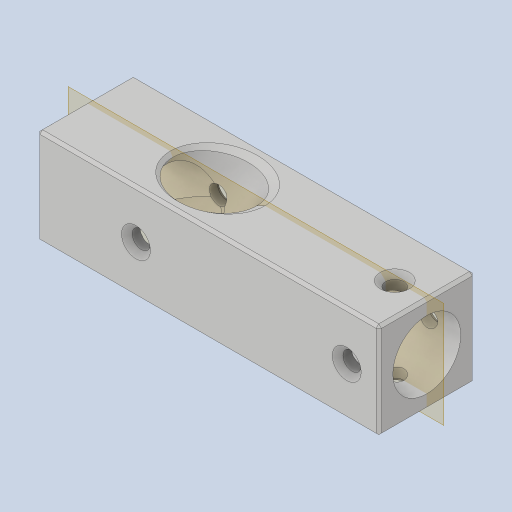
# Autodesk Inventor part: holderHolder
Saved by Autodesk Inventor 2024.1 (Build 281209000, 209)
## iProperties
Created: 2019-08-19
Part Number: holderHolder
Material: Generic
Document SubType Name: Modeling
Designer: Daniel
Density: 1 g/cm^3
Appearance: Default
Author: Daniel
Autodesk Inventor part; units mm, degrees
sketch "Sketch1" plane through (0, 0, 0) normal (0, 1, 0) x (-1, 0, 0)
  line L0 (0, 0) -> (-60, 0)
  line L1 (-60, 0) -> (-60, -18)
  line L2 (-60, -18) -> (0, -18)
  line L3 (0, -18) -> (0, 0)
  dimension "d0" = 60
  dimension "d1" = 18
  constraints: 8 end point, 2 parallel, 1 horizontal, 1 perpendicular
  measures "d0" distance of L1.end L2.end
  measures "d1" distance of L2.end L0.start
extrude "Extrusion1" add sketch "Sketch1" along normal blind 18
sketch "Sketch2" plane through (60, 0, 0) normal (1, 0, 0) x (0, 0, -1)
  line L0 (14.7, 6.639) -> (11.361, 3.3)
  line L1 (11.361, 3.3) -> (6.639, 3.3)
  line L2 (6.639, 3.3) -> (3.3, 6.639)
  line L3 (3.3, 6.639) -> (3.3, 11.361)
  line L4 (3.3, 11.361) -> (6.639, 14.7)
  line L5 (6.639, 14.7) -> (11.361, 14.7)
  line L6 (11.361, 14.7) -> (14.7, 11.361)
  line L7 (14.7, 11.361) -> (14.7, 6.639)
  line L8 (0, 18) -> (18, 18) construction
  line L9 (9, 18) -> (9, 0) construction
  line L10 (0, 0) -> (18, 0) construction
  line L11 (0, 0) -> (0, 18) construction
  line L12 (0, 9) -> (18, 9) construction
  line L13 (18, 0) -> (18, 18) construction
  point P0 (9, 9)
  dimension "d4" = 11.4
  dimension "d28" = 0
  constraints: 20 end point, 5 midpoint, 17 other
  measures "d4" distance between parallel lines of L1 L5
  measures "d28" angle of L12 L5
extrude "Extrusion2" cut sketch "Sketch2" against normal blind 18
sketch "Sketch3" plane through (42, 0, 0) normal (1, 0, 0) x (0, 0, -1)
  line L0 (14.7, 6.639) -> (11.361, 3.3) projected
  line L1 (14.7, 11.361) -> (14.7, 6.639) projected
  line L2 (11.361, 14.7) -> (14.7, 11.361) projected
  line L3 (6.639, 14.7) -> (11.361, 14.7) projected
  line L4 (3.3, 11.361) -> (6.639, 14.7) projected
  line L5 (3.3, 6.639) -> (3.3, 11.361) projected
  line L6 (6.639, 3.3) -> (3.3, 6.639) projected
  line L7 (11.361, 3.3) -> (6.639, 3.3) projected
  circle A0 centre (9, 9) radius 4
  point P0 (0, 0)
  dimension "d7" = 8
  constraints: 1 centre point
  measures "d7" diameter of A0
extrude "Extrusion3" cut sketch "Sketch3" against normal through all contours A0
sketch "Sketch4" plane through (0, 0, -18) normal (-1, 0, 0) x (0, 0, 1)
  circle A0 centre (9, 9) radius 4 projected
  circle A1 centre (9, 9) radius 6.5
  point P0 (18, 0)
  dimension "d10" = 13
  constraints: 1 centre point, 1 coincident
  measures "d10" diameter of A1
extrude "Extrusion4" cut sketch "Sketch4" against normal blind 20
ref_plane "Work Plane1" through (0, 0, -18) normal (-0.5735764, -0.819152, 0) x (0, 0, 1)
sketch "Sketch5" plane through (-5.043, 3.5311, 0) normal (0.5735764, 0.819152, 0) x (0.819152, -0.5735764, 0)
  circle A0 centre (16.1564, 9) radius 6.45
  line L0 (6.1564, 18) -> (6.1564, 0) construction
  line L1 (6.1564, 9) -> (16.1564, 9) construction
  dimension "d13" = 12.9
  dimension "d27" = 10
  constraints: 2 end point, 1 centre point, 1 horizontal, 1 midpoint
  measures "d13" diameter of A0
  measures "d27" distance from line of L0 L1.end
extrude "Extrusion5" cut sketch "Sketch5" along normal through all
ref_plane "Work Plane3" through (0, 0, -18) normal (0, -1, 0) x (0, 0, 1)
ref_plane "Work Plane2" through (42, -7.45, -11.361) normal (0, 1, 0) x (1, 0, 0)
sketch "Sketch9" plane through (60, 0, 0) normal (1, 0, 0) x (0, 0, -1)
  arc A0 (2.5812, 10.0241) -> (15.4188, 10.0241) centre (9, 9) ccw projected
  circle A1 centre (9, 9) radius 6
  line L0 (0, 0) -> (0, 18) projected
  line L1 (0, 18) -> (18, 18) projected
  line L2 (0, 0) -> (18, 0) projected
  line L3 (18, 0) -> (18, 18) projected
  dimension "d49" = 12
  constraints: 1 centre point, 1 coincident
  measures "d49" diameter of A1
extrude "Extrusion9" add sketch "Sketch9" along normal blind 4
sketch "Sketch6" plane through (0, 0, 0) normal (0, 0, 1) x (1, 0, 0)
  line L0 (0, 0) -> (0, 18) construction
  line L1 (0, 9) -> (48.5921, 9) construction
  circle A0 centre (18.5096, 9) radius 1.7
  line L2 (20.0817, 0) -> (4.3337, 0) projected
  line L3 (16.9375, 18) -> (32.6855, 18) projected
  line L4 (16.9375, 18) -> (20.0817, 0) construction
  line L5 (32.6855, 18) -> (4.3337, 0) construction
  dimension "d23" = 3.4
  constraints: 6 end point, 2 midpoint, 1 centre point, 1 point on line
  measures "d23" diameter of A0
extrude "Extrusion6" cut sketch "Sketch6" against normal through all
sketch "Sketch10" plane through (0, 0, -18) normal (0, -1, 0) x (0, 0, 1)
  circle A0 centre (9, -18.5096) radius 6.45
  line L0 (0, 0) -> (18, 0) projected
  line L1 (18, -16.8096) -> (18, -20.2096) projected
  point P0 (9, 0)
  point P1 (9, 0)
  point P2 (18, -18.5096)
  dimension "d59" = 12.9
  constraints: 3 midpoint, 2 vertical alignment, 1 centre point, 1 horizontal alignment
  measures "d59" diameter of A0
extrude "Extrusion10" [suppressed]
sketch "Sketch7" plane through (42, -7.45, -11.361) normal (0, 1, 0) x (1, 0, 0)
  circle A0 centre (16, -2.361) radius 1.7
  line L0 (18, -0.4875) -> (18, -4.2345) projected
  line L1 (18, 0) -> (0, 0) projected
  line L2 (0, 0) -> (0, -4.722) projected
  line L3 (18, -4.722) -> (0, -4.722) projected
  line L4 (18, 0) -> (18, -0.4875) projected
  line L5 (18, -4.2345) -> (18, -4.722) projected
  point P0 (-42, -11.361)
  dimension "d30" = 3.4
  dimension "d31" = 2.361
  dimension "d32" = 2.361
  dimension "d33" = 2
  constraints: 1 centre point
  measures "d30" diameter of A0
  measures "d31" distance from line of L1 A0.centre
  measures "d32" distance from line of L3 A0.centre
  measures "d33" distance from line of L0 A0.centre
extrude "Extrusion7" cut sketch "Sketch7" along normal through all contours A0
pattern_circular "Circular Pattern1" count 4 over 360 about axis through (60, 9, -9) along (1, 0, 0) of "Extrusion7"
ref_plane "Work Plane4" through (0, 0, -9) normal (0, 0, 1) x (1, 0, 0)
sketch "Sketch8" plane through (0, 0, 0) normal (0, -1, 0) x (1, 0, 0)
  line L0 (32, -18) -> (46, -18) construction
  line L1 (46, -18) -> (46, 0) construction
  line L2 (46, 0) -> (32, 0) construction
  line L3 (32, 0) -> (32, -18) construction
  line L4 (0, 0) -> (64, 0) projected
  line L5 (0, 0) -> (64, 0) projected
  line L6 (0, -18) -> (64, -18) projected
  circle A0 centre (58, -9) radius 1.7 projected
  spline S0 degree 2 poles (35.027, -5.8856) (35.027, -6.0832) (34.8862, -6.4389) (34.7602, -6.5624) knots 0 0 0 1 2 2 2
  spline S1 degree 2 poles (34.7602, -6.5624) (34.6021, -6.718) (34.1748, -6.8786) (33.8488, -6.8786) knots 0 0 0 1 2 2 2
  line L7 (33.8488, -6.8786) -> (33.5054, -6.8786)
  line L8 (33.5054, -6.8786) -> (33.5054, -8.0148)
  line L9 (33.5054, -8.0148) -> (33.1004, -8.0148)
  line L10 (33.1004, -8.0148) -> (33.1004, -4.9668)
  line L11 (33.1004, -4.9668) -> (33.8661, -4.9668)
  spline S2 degree 2 poles (33.8661, -4.9668) (34.1378, -4.9668) (34.5182, -5.0557) (34.6639, -5.157) knots 0 0 0 1 2 2 2
  spline S3 degree 2 poles (34.6639, -5.157) (34.8343, -5.2731) (35.027, -5.6312) (35.027, -5.8856) knots 0 0 0 1 2 2 2
  spline S4 degree 2 poles (34.6046, -5.898) (34.6046, -5.7399) (34.4959, -5.5077) (34.3848, -5.4336) knots 0 0 0 1 2 2 2
  spline S5 degree 2 poles (34.3848, -5.4336) (34.2884, -5.3694) (34.0316, -5.3175) (33.8414, -5.3175) knots 0 0 0 1 2 2 2
  line L12 (33.8414, -5.3175) -> (33.5054, -5.3175)
  line L13 (33.5054, -5.3175) -> (33.5054, -6.5328)
  line L14 (33.5054, -6.5328) -> (33.7821, -6.5328)
  spline S6 degree 2 poles (33.7821, -6.5328) (34.0291, -6.5328) (34.3329, -6.4537) (34.4317, -6.35) knots 0 0 0 1 2 2 2
  spline S7 degree 2 poles (34.4317, -6.35) (34.5231, -6.2586) (34.6046, -6.0437) (34.6046, -5.898) knots 0 0 0 1 2 2 2
  spline S8 degree 2 poles (36.1484, -5.2558) (36.0372, -5.2558) (35.8174, -5.3101) (35.7112, -5.3521) knots 0 0 0 1 2 2 2
  spline S9 degree 2 poles (35.7112, -5.3521) (35.6124, -5.3941) (35.4666, -5.483) (35.4098, -5.5225) knots 0 0 0 1 2 2 2
  line L15 (35.4098, -5.5225) -> (35.3851, -5.5225)
  line L16 (35.3851, -5.5225) -> (35.3851, -5.0903)
  spline S10 degree 2 poles (35.3851, -5.0903) (35.5185, -5.0186) (35.9755, -4.9026) (36.1805, -4.9026) knots 0 0 0 1 2 2 2
  spline S11 degree 2 poles (36.1805, -4.9026) (36.388, -4.9026) (36.6967, -4.9865) (36.8227, -5.0755) knots 0 0 0 1 2 2 2
  spline S12 degree 2 poles (36.8227, -5.0755) (36.9561, -5.1718) (37.0944, -5.4509) (37.0944, -5.6386) knots 0 0 0 1 2 2 2
  spline S13 degree 2 poles (37.0944, -5.6386) (37.0944, -5.8906) (36.7634, -6.2709) (36.5312, -6.3203) knots 0 0 0 1 2 2 2
  line L17 (36.5312, -6.3203) -> (36.5312, -6.35)
  spline S14 degree 2 poles (36.5312, -6.35) (36.6275, -6.3697) (36.8474, -6.4587) (36.9412, -6.5476) knots 0 0 0 1 2 2 2
  spline S15 degree 2 poles (36.9412, -6.5476) (37.0351, -6.634) (37.1537, -6.9107) (37.1537, -7.1107) knots 0 0 0 1 2 2 2
  spline S16 degree 2 poles (37.1537, -7.1107) (37.1537, -7.3158) (37.0129, -7.664) (36.8844, -7.7974) knots 0 0 0 1 2 2 2
  spline S17 degree 2 poles (36.8844, -7.7974) (36.7511, -7.9357) (36.3731, -8.079) (36.1335, -8.079) knots 0 0 0 1 2 2 2
  spline S18 degree 2 poles (36.1335, -8.079) (35.9038, -8.079) (35.4543, -7.9678) (35.3012, -7.8913) knots 0 0 0 1 2 2 2
  line L18 (35.3012, -7.8913) -> (35.3012, -7.459)
  line L19 (35.3012, -7.459) -> (35.3308, -7.459)
  spline S19 degree 2 poles (35.3308, -7.459) (35.4592, -7.5529) (35.894, -7.7258) (36.1088, -7.7258) knots 0 0 0 1 2 2 2
  spline S20 degree 2 poles (36.1088, -7.7258) (36.2348, -7.7258) (36.4868, -7.6467) (36.5707, -7.5554) knots 0 0 0 1 2 2 2
  spline S21 degree 2 poles (36.5707, -7.5554) (36.6522, -7.464) (36.7387, -7.2466) (36.7387, -7.0811) knots 0 0 0 1 2 2 2
  spline S22 degree 2 poles (36.7387, -7.0811) (36.7387, -6.9156) (36.6424, -6.7007) (36.5559, -6.639) knots 0 0 0 1 2 2 2
  spline S23 degree 2 poles (36.5559, -6.639) (36.4695, -6.5772) (36.2348, -6.5303) (36.0965, -6.5303) knots 0 0 0 1 2 2 2
  line L20 (36.0965, -6.5303) -> (35.9236, -6.5303)
  line L21 (35.9236, -6.5303) -> (35.9236, -6.1919)
  line L22 (35.9236, -6.1919) -> (36.0594, -6.1919)
  spline S24 degree 2 poles (36.0594, -6.1919) (36.3336, -6.1919) (36.6794, -5.9301) (36.6794, -5.6806) knots 0 0 0 1 2 2 2
  spline S25 degree 2 poles (36.6794, -5.6806) (36.6794, -5.5645) (36.5905, -5.399) (36.5189, -5.3496) knots 0 0 0 1 2 2 2
  spline S26 degree 2 poles (36.5189, -5.3496) (36.4423, -5.2978) (36.2546, -5.2558) (36.1484, -5.2558) knots 0 0 0 1 2 2 2
  spline S27 degree 2 poles (39.4607, -7.0465) (39.4607, -7.2664) (39.3199, -7.6418) (39.1914, -7.7801) knots 0 0 0 1 2 2 2
  spline S28 degree 2 poles (39.1914, -7.7801) (39.063, -7.9184) (38.6801, -8.079) (38.443, -8.079) knots 0 0 0 1 2 2 2
  spline S29 degree 2 poles (38.443, -8.079) (38.2256, -8.079) (37.8008, -7.9827) (37.6452, -7.9061) knots 0 0 0 1 2 2 2
  line L23 (37.6452, -7.9061) -> (37.6452, -7.4738)
  line L24 (37.6452, -7.4738) -> (37.6748, -7.4738)
  spline S30 degree 2 poles (37.6748, -7.4738) (37.7218, -7.5084) (37.8971, -7.5973) (38.0033, -7.6369) knots 0 0 0 1 2 2 2
  spline S31 degree 2 poles (38.0033, -7.6369) (38.1244, -7.6789) (38.3245, -7.7258) (38.4504, -7.7258) knots 0 0 0 1 2 2 2
  spline S32 degree 2 poles (38.4504, -7.7258) (38.5739, -7.7258) (38.8061, -7.6369) (38.8901, -7.5405) knots 0 0 0 1 2 2 2
  spline S33 degree 2 poles (38.8901, -7.5405) (38.9667, -7.4491) (39.0457, -7.2071) (39.0457, -7.0441) knots 0 0 0 1 2 2 2
  spline S34 degree 2 poles (39.0457, -7.0441) (39.0457, -6.881) (38.9568, -6.6736) (38.8728, -6.6044) knots 0 0 0 1 2 2 2
  spline S35 degree 2 poles (38.8728, -6.6044) (38.7863, -6.5278) (38.5295, -6.4636) (38.3739, -6.4636) knots 0 0 0 1 2 2 2
  spline S36 degree 2 poles (38.3739, -6.4636) (38.2059, -6.4636) (37.8724, -6.5155) (37.7712, -6.5377) knots 0 0 0 1 2 2 2
  line L25 (37.7712, -6.5377) -> (37.7712, -4.9668)
  line L26 (37.7712, -4.9668) -> (39.4434, -4.9668)
  line L27 (39.4434, -4.9668) -> (39.4434, -5.3249)
  line L28 (39.4434, -5.3249) -> (38.1639, -5.3249)
  line L29 (38.1639, -5.3249) -> (38.1639, -6.1376)
  spline S37 degree 2 poles (38.1639, -6.1376) (38.238, -6.1277) (38.3813, -6.1203) (38.4405, -6.1203) knots 0 0 0 1 2 2 2
  spline S38 degree 2 poles (38.4405, -6.1203) (38.6752, -6.1203) (38.9988, -6.1968) (39.147, -6.3105) knots 0 0 0 1 2 2 2
  spline S39 degree 2 poles (39.147, -6.3105) (39.2976, -6.4241) (39.4607, -6.7699) (39.4607, -7.0465) knots 0 0 0 1 2 2 2
  line L30 (40.5549, -8.0148) -> (40.0658, -8.0148)
  line L31 (40.0658, -8.0148) -> (40.0658, -7.4319)
  line L32 (40.0658, -7.4319) -> (40.5549, -7.4319)
  line L33 (40.5549, -7.4319) -> (40.5549, -8.0148)
  spline S40 degree 2 poles (43.0669, -6.4908) (43.0669, -7.3108) (42.5902, -8.079) (42.0937, -8.079) knots 0 0 0 1 2 2 2
  spline S41 degree 2 poles (42.0937, -8.079) (41.5898, -8.079) (41.118, -7.296) (41.118, -6.4932) knots 0 0 0 1 2 2 2
  spline S42 degree 2 poles (41.118, -6.4932) (41.118, -5.6683) (41.5948, -4.905) (42.0937, -4.905) knots 0 0 0 1 2 2 2
  spline S43 degree 2 poles (42.0937, -4.905) (42.5951, -4.905) (43.0669, -5.6954) (43.0669, -6.4908) knots 0 0 0 1 2 2 2
  spline S44 degree 2 poles (42.5432, -7.4195) (42.6025, -7.2688) (42.6519, -6.8045) (42.6519, -6.4908) knots 0 0 0 1 2 2 2
  spline S45 degree 2 poles (42.6519, -6.4908) (42.6519, -6.1771) (42.6025, -5.7152) (42.5408, -5.5596) knots 0 0 0 1 2 2 2
  spline S46 degree 2 poles (42.5408, -5.5596) (42.479, -5.404) (42.2641, -5.2434) (42.0937, -5.2434) knots 0 0 0 1 2 2 2
  spline S47 degree 2 poles (42.0937, -5.2434) (41.9233, -5.2434) (41.7034, -5.404) (41.6392, -5.5645) knots 0 0 0 1 2 2 2
  spline S48 degree 2 poles (41.6392, -5.5645) (41.5775, -5.7201) (41.533, -6.1944) (41.533, -6.4932) knots 0 0 0 1 2 2 2
  spline S49 degree 2 poles (41.533, -6.4932) (41.533, -6.8143) (41.5725, -7.2441) (41.6367, -7.4121) knots 0 0 0 1 2 2 2
  spline S50 degree 2 poles (41.6367, -7.4121) (41.696, -7.5702) (41.9159, -7.7406) (42.0937, -7.7406) knots 0 0 0 1 2 2 2
  spline S51 degree 2 poles (42.0937, -7.7406) (42.2617, -7.7406) (42.4815, -7.5801) (42.5432, -7.4195) knots 0 0 0 1 2 2 2
  spline S52 degree 2 poles (45.0009, -5.693) (45.0009, -6.0215) (44.5514, -6.471) (44.2228, -6.471) knots 0 0 0 1 2 2 2
  spline S53 degree 2 poles (44.2228, -6.471) (43.8968, -6.471) (43.4423, -6.0239) (43.4423, -5.693) knots 0 0 0 1 2 2 2
  spline S54 degree 2 poles (43.4423, -5.693) (43.4423, -5.3644) (43.8919, -4.9149) (44.2228, -4.9149) knots 0 0 0 1 2 2 2
  spline S55 degree 2 poles (44.2228, -4.9149) (44.5514, -4.9149) (45.0009, -5.3644) (45.0009, -5.693) knots 0 0 0 1 2 2 2
  spline S56 degree 2 poles (44.6798, -5.693) (44.6798, -5.4954) (44.418, -5.2261) (44.2228, -5.2261) knots 0 0 0 1 2 2 2
  spline S57 degree 2 poles (44.2228, -5.2261) (44.0252, -5.2261) (43.7634, -5.4954) (43.7634, -5.693) knots 0 0 0 1 2 2 2
  spline S58 degree 2 poles (43.7634, -5.693) (43.7634, -5.893) (44.0302, -6.1598) (44.2228, -6.1598) knots 0 0 0 1 2 2 2
  spline S59 degree 2 poles (44.2228, -6.1598) (44.418, -6.1598) (44.6798, -5.8881) (44.6798, -5.693) knots 0 0 0 1 2 2 2
  line L34 (36.4584, -13.0332) -> (35.9322, -13.0332)
  line L35 (35.9322, -13.0332) -> (34.9689, -11.8204)
  line L36 (34.9689, -11.8204) -> (34.5046, -11.8204)
  line L37 (34.5046, -11.8204) -> (34.5046, -13.0332)
  line L38 (34.5046, -13.0332) -> (34.0995, -13.0332)
  line L39 (34.0995, -13.0332) -> (34.0995, -9.9852)
  line L40 (34.0995, -9.9852) -> (34.885, -9.9852)
  spline S60 degree 2 poles (34.885, -9.9852) (35.1468, -9.9852) (35.5, -10.042) (35.6605, -10.1458) knots 0 0 0 1 2 2 2
  spline S61 degree 2 poles (35.6605, -10.1458) (35.8211, -10.2495) (36.0063, -10.5731) (36.0063, -10.8127) knots 0 0 0 1 2 2 2
  spline S62 degree 2 poles (36.0063, -10.8127) (36.0063, -11.1461) (35.6655, -11.5981) (35.374, -11.7068) knots 0 0 0 1 2 2 2
  line L41 (35.374, -11.7068) -> (36.4584, -13.0332)
  spline S63 degree 2 poles (35.584, -10.8448) (35.584, -10.7114) (35.4901, -10.5064) (35.3913, -10.4397) knots 0 0 0 1 2 2 2
  spline S64 degree 2 poles (35.3913, -10.4397) (35.3049, -10.3829) (35.0751, -10.336) (34.9072, -10.336) knots 0 0 0 1 2 2 2
  line L42 (34.9072, -10.336) -> (34.5046, -10.336)
  line L43 (34.5046, -10.336) -> (34.5046, -11.4821)
  line L44 (34.5046, -11.4821) -> (34.8603, -11.4821)
  spline S65 degree 2 poles (34.8603, -11.4821) (35.0356, -11.4821) (35.3147, -11.4203) (35.4111, -11.324) knots 0 0 0 1 2 2 2
  spline S66 degree 2 poles (35.4111, -11.324) (35.5, -11.24) (35.584, -11.0029) (35.584, -10.8448) knots 0 0 0 1 2 2 2
  spline S67 degree 2 poles (38.5109, -11.5092) (38.5109, -12.3293) (38.0342, -13.0974) (37.5378, -13.0974) knots 0 0 0 1 2 2 2
  spline S68 degree 2 poles (37.5378, -13.0974) (37.0339, -13.0974) (36.5621, -12.3145) (36.5621, -11.5117) knots 0 0 0 1 2 2 2
  spline S69 degree 2 poles (36.5621, -11.5117) (36.5621, -10.6867) (37.0388, -9.9235) (37.5378, -9.9235) knots 0 0 0 1 2 2 2
  spline S70 degree 2 poles (37.5378, -9.9235) (38.0392, -9.9235) (38.5109, -10.7139) (38.5109, -11.5092) knots 0 0 0 1 2 2 2
  spline S71 degree 2 poles (37.9873, -12.438) (38.0466, -12.2873) (38.096, -11.8229) (38.096, -11.5092) knots 0 0 0 1 2 2 2
  spline S72 degree 2 poles (38.096, -11.5092) (38.096, -11.1955) (38.0466, -10.7336) (37.9848, -10.578) knots 0 0 0 1 2 2 2
  spline S73 degree 2 poles (37.9848, -10.578) (37.9231, -10.4224) (37.7082, -10.2619) (37.5378, -10.2619) knots 0 0 0 1 2 2 2
  spline S74 degree 2 poles (37.5378, -10.2619) (37.3673, -10.2619) (37.1475, -10.4224) (37.0833, -10.583) knots 0 0 0 1 2 2 2
  spline S75 degree 2 poles (37.0833, -10.583) (37.0215, -10.7386) (36.9771, -11.2128) (36.9771, -11.5117) knots 0 0 0 1 2 2 2
  spline S76 degree 2 poles (36.9771, -11.5117) (36.9771, -11.8328) (37.0166, -12.2626) (37.0808, -12.4305) knots 0 0 0 1 2 2 2
  spline S77 degree 2 poles (37.0808, -12.4305) (37.1401, -12.5886) (37.3599, -12.7591) (37.5378, -12.7591) knots 0 0 0 1 2 2 2
  spline S78 degree 2 poles (37.5378, -12.7591) (37.7057, -12.7591) (37.9255, -12.5985) (37.9873, -12.438) knots 0 0 0 1 2 2 2
  line L45 (39.5558, -13.0332) -> (39.0667, -13.0332)
  line L46 (39.0667, -13.0332) -> (39.0667, -12.4503)
  line L47 (39.0667, -12.4503) -> (39.5558, -12.4503)
  line L48 (39.5558, -12.4503) -> (39.5558, -13.0332)
  spline S79 degree 2 poles (42.0678, -11.5092) (42.0678, -12.3293) (41.591, -13.0974) (41.0946, -13.0974) knots 0 0 0 1 2 2 2
  spline S80 degree 2 poles (41.0946, -13.0974) (40.5907, -13.0974) (40.1189, -12.3145) (40.1189, -11.5117) knots 0 0 0 1 2 2 2
  spline S81 degree 2 poles (40.1189, -11.5117) (40.1189, -10.6867) (40.5956, -9.9235) (41.0946, -9.9235) knots 0 0 0 1 2 2 2
  spline S82 degree 2 poles (41.0946, -9.9235) (41.596, -9.9235) (42.0678, -10.7139) (42.0678, -11.5092) knots 0 0 0 1 2 2 2
  spline S83 degree 2 poles (41.5441, -12.438) (41.6034, -12.2873) (41.6528, -11.8229) (41.6528, -11.5092) knots 0 0 0 1 2 2 2
  spline S84 degree 2 poles (41.6528, -11.5092) (41.6528, -11.1955) (41.6034, -10.7336) (41.5416, -10.578) knots 0 0 0 1 2 2 2
  spline S85 degree 2 poles (41.5416, -10.578) (41.4799, -10.4224) (41.265, -10.2619) (41.0946, -10.2619) knots 0 0 0 1 2 2 2
  spline S86 degree 2 poles (41.0946, -10.2619) (40.9241, -10.2619) (40.7043, -10.4224) (40.6401, -10.583) knots 0 0 0 1 2 2 2
  spline S87 degree 2 poles (40.6401, -10.583) (40.5783, -10.7386) (40.5339, -11.2128) (40.5339, -11.5117) knots 0 0 0 1 2 2 2
  spline S88 degree 2 poles (40.5339, -11.5117) (40.5339, -11.8328) (40.5734, -12.2626) (40.6376, -12.4305) knots 0 0 0 1 2 2 2
  spline S89 degree 2 poles (40.6376, -12.4305) (40.6969, -12.5886) (40.9167, -12.7591) (41.0946, -12.7591) knots 0 0 0 1 2 2 2
  spline S90 degree 2 poles (41.0946, -12.7591) (41.2625, -12.7591) (41.4824, -12.5985) (41.5441, -12.438) knots 0 0 0 1 2 2 2
  spline S91 degree 2 poles (44.0018, -10.7114) (44.0018, -11.0399) (43.5522, -11.4895) (43.2237, -11.4895) knots 0 0 0 1 2 2 2
  spline S92 degree 2 poles (43.2237, -11.4895) (42.8977, -11.4895) (42.4432, -11.0424) (42.4432, -10.7114) knots 0 0 0 1 2 2 2
  spline S93 degree 2 poles (42.4432, -10.7114) (42.4432, -10.3829) (42.8927, -9.9334) (43.2237, -9.9334) knots 0 0 0 1 2 2 2
  spline S94 degree 2 poles (43.2237, -9.9334) (43.5522, -9.9334) (44.0018, -10.3829) (44.0018, -10.7114) knots 0 0 0 1 2 2 2
  spline S95 degree 2 poles (43.6807, -10.7114) (43.6807, -10.5138) (43.4189, -10.2446) (43.2237, -10.2446) knots 0 0 0 1 2 2 2
  spline S96 degree 2 poles (43.2237, -10.2446) (43.0261, -10.2446) (42.7643, -10.5138) (42.7643, -10.7114) knots 0 0 0 1 2 2 2
  spline S97 degree 2 poles (42.7643, -10.7114) (42.7643, -10.9115) (43.0311, -11.1782) (43.2237, -11.1782) knots 0 0 0 1 2 2 2
  spline S98 degree 2 poles (43.2237, -11.1782) (43.4189, -11.1782) (43.6807, -10.9065) (43.6807, -10.7114) knots 0 0 0 1 2 2 2
  point P0 (60, 0)
  dimension "roll" = 0
  dimension "pitch" = 35
  dimension "d53" = 14
  dimension "d68" = 12
  constraints: 2 collinear, 2 other
  measures "d53" distance between parallel lines of L1 L3
  measures "d68" distance from line of A0.centre L1
extrude "Extrusion8" cut sketch "Sketch8" against normal blind 0.75 contours S0 S1 L7 L8 L9 L10 L11 S2 S3 | S8 S9 L15 L16 S10 S11 S12 S13 L17 S14 S15 S16 S17 S18 L18 L19 S19 S20 S21 S22 S23 L20 L21 L22 S24 S25 S26 | S27 S28 S29 L23 L24 S30 S31 S32 S33 S34 S35 S36 L25 L26 L27 L28 L29 S37 S38 S39 | L30 L31 L32 L33 | S40 S41 S42 S43 | S52 S53 S54 S55 | L34 L35 L36 L37 L38 L39 L40 S60 S61 S62 L41 | S67 S68 S69 S70 | L45 L46 L47 L48 | S79 S80 S81 S82 | S91 S92 S93 S94
sketch "Sketch11" plane through (64, 0, 0) normal (1, 0, 0) x (0, 0, -1)
  line L0 (18, 0) -> (0, 0) projected
  line L1 (18, 0) -> (23.25, 0)
  line L2 (23.25, 0) -> (23.25, 2)
  line L3 (23.25, 2) -> (18, 2)
  line L4 (18, 2) -> (18, 0)
  line L5 (23.25, 2) -> (21.25, 2)
  line L6 (21.25, 2) -> (21.25, 8)
  line L7 (21.25, 8) -> (23.25, 8)
  line L8 (23.25, 8) -> (23.25, 2)
  line L9 (18, 0) -> (18, 18) projected
  line L10 (18, 18) -> (0, 18) projected
  dimension "d63" = 3.25
  dimension "d64" = 2
  dimension "d65" = 2
  dimension "d69" = 6
  constraints: 16 end point, 4 parallel, 2 horizontal, 2 perpendicular
  measures "d63" distance between parallel lines of L6 L9
  measures "d64" distance of L1.end L2.end
  measures "d65" distance of L6.end L7.end
  measures "d69" distance between parallel lines of L3 L7
extrude "Extrusion11" [suppressed]
sketch "Sketch13" plane through (64, 0, -23.25) normal (0, 0, -1) x (-1, 0, 0)
  circle A0 centre (6, 9) radius 1.7 construction
  circle A1 centre (43.394, 9) radius 1.7 construction
  circle A2 centre (6, 9) radius 4
  circle A3 centre (43.394, 9) radius 1.7 projected
  circle A4 centre (43.394, 9) radius 4
  point P0 (64, 0)
  dimension "d70" = 8
  constraints: 2 centre point, 2 coincident, 1 equal radius
  measures "d70" diameter of A2
extrude "Extrusion12" [suppressed]
mirror "Mirror1" [suppressed]
chamfer "Chamfer2" distance 0.5 angle 45 9 edges at (32, 18, 0) (32, 18, -18) (0, 9, -18) (0, 0, -9) (0, 9, 0) (0, 18, -9) (64, 18, -9) (64, 9, 0) (64, 9, -18)
chamfer "Chamfer3" distance 1 angle 45 9 edges at (16.8096, 9, 0) (16.8096, 9, -18) (56.3, 0, -9) (56.3, 18, -9) (0, 9, -15.5) (16.9375, 18, -9) (4.3337, 0, -9) (56.3, 9, 0) (56.3, 9, -18)
chamfer "Chamfer4" distance 0.5 angle 45 3 edges at (32, 0, 0) (32, 0, -18) (64, 0, -9)
sketch "Sketch14" plane through (64, 0, 0) normal (1, 0, 0) x (0, 0, -1)
  circle A0 centre (9, 9) radius 6 projected
  circle A1 centre (9, 9) radius 6.35
  point P0 (0, 0)
  dimension "d77" = 12.7
  constraints: 1 centre point, 1 coincident
  measures "d77" diameter of A1
extrude "Extrusion13" cut sketch "Sketch14" against normal up to surface (22 mm away) contours A0 | A1
equation "\"d31\" = d32"
equation "\"roll\" = 0"
equation "\"pitch\" = 35deg"
equation "\"d25\" = -pitch"
equation "\"pitch2\" = 0"
body "Solid1"
